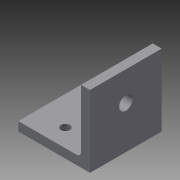
# Autodesk Inventor part: clevece plate
Saved by Autodesk Inventor 2015 (Build 190159000, 159)
## iProperties
Created: 2015-02-04
Part Number: clevece plate
Material: Generic
Document SubType Name: Modeling
Designer: mastkee16
Density: 1 g/cm^3
Appearance: Default
Author: mastkee16
Autodesk Inventor part; units mm, degrees
ref_plane "YZ Plane" through (0, 0, 0) normal (1, 0, 0) x (0, 1, 0)
ref_plane "XZ Plane" through (0, 0, 0) normal (0, 1, 0) x (-1, 0, 0)
ref_plane "XY Plane" through (0, 0, 0) normal (0, 0, 1) x (1, 0, 0)
sketch "Sketch1" plane through (0, 0, 0) normal (0, 0, 1) x (1, 0, 0)
  line L0 (0, 0) -> (50.8, 0)
  line L1 (50.8, 0) -> (50.8, 50.8)
  line L2 (50.8, 50.8) -> (0, 50.8)
  line L3 (0, 50.8) -> (0, 0)
  dimension "d0" = 50.8
  dimension "d1" = 50.8
  constraints: 8 end point, 2 parallel, 1 horizontal, 1 perpendicular
  measures "d0" distance of L2.end L1.end
  measures "d1" distance of L1.end L0.end
extrude "Extrusion1" add sketch "Sketch1" along normal blind 50.8
sketch "Sketch2" plane through (0, 0, 50.8) normal (0, 0, 1) x (1, 0, 0)
  line L0 (0, 50.8) -> (44.45, 50.8)
  line L1 (44.45, 50.8) -> (44.45, 6.35)
  line L2 (44.45, 6.35) -> (0, 6.35)
  line L3 (0, 6.35) -> (0, 50.8)
  point P0 (0, 0)
  dimension "d4" = 44.45
  dimension "d5" = 44.45
  constraints: 8 end point, 2 parallel, 1 horizontal, 1 perpendicular
  measures "d4" distance of L1.end L2.end
  measures "d5" distance of L0.end L1.end
extrude "Extrusion2" cut sketch "Sketch2" against normal blind 152.4
fillet "Fillet1" radius 3.175 1 edges at (44.45, 6.35, 25.4)
sketch "Sketch3" plane through (44.45, 50.8, 0) normal (-1, 0, 0) x (0, 0, 1)
  circle A0 centre (25.4, -20.6375) radius 4.7625
  line L0 (0, -41.275) -> (0, 0) projected
  line L1 (0, 0) -> (50.8, 0) projected
  point P0 (0, -50.8)
  dimension "d9" = 9.525
  dimension "d10" = 25.4
  dimension "d11" = 20.6375
  constraints: 1 centre point
  measures "d9" diameter of A0
  measures "d10" distance from line of L0 A0.centre
  measures "d11" distance from line of A0.centre L1
extrude "Extrusion3" cut sketch "Sketch3" against normal blind 152.4
sketch "Sketch4" plane through (0, 6.35, 50.8) normal (0, 1, 0) x (1, 0, 0)
  line L0 (0, 50.8) -> (41.275, 50.8) projected
  line L1 (0, 0) -> (0, 50.8) projected
  point P0 (20.6375, 38.1)
  point P1 (20.6375, 12.7)
  dimension "d14" = 25.4
  dimension "d15" = 12.7
  dimension "d16" = 20.6375
  dimension "d17" = 20.6375
  measures "d14" distance of point (20.638, 12.7) point (20.638, 38.1)
  measures "d15" distance from line of point (20.638, 38.1) L0
  measures "d16" distance from line of point (20.638, 38.1) L1
  measures "d17" distance from line of point (20.638, 12.7) L1
hole "Hole1" at (20.6375, 6.35, 12.7) at (20.6375, 6.35, 38.1) direction (0, -1, 0) diameter 6.35 end through all
body "Solid1"
